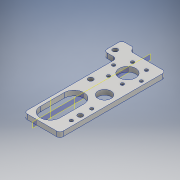
# Autodesk Inventor part: side_plate
Saved by Autodesk Inventor 2018 (Build 220112000, 112)
## iProperties
Created: 2019-01-31
Part Number: side_plate
Material: Aluminum 6061
Document SubType Name: Modeling
Designer: steve
Density: 2.7 g/cm^3
Appearance: Aluminum - Flat
Mass: 11.8642 g
Surface Area: 37.8269 cm^2
Volume: 4.39413 cm^3
d0: 10,000 mm
d1: 10,100 mm
d2: 25,000 mm
d3: 13,000 mm
d4: 15,000 mm
d5: 8,000 mm
d6: 42,800 mm
d7: 45,00 deg
d8: 38,100 mm
d9: 6,000 mm
d10: 2,000 mm
d11: 3,000 mm
d12: 3,000 mm
d13: 3,000 mm
d14: 0,00 deg
d15: 17,000 mm
d16: 6,000 ul
d20: 2,000 mm
d27: 22,000 mm
d28: 12,100 mm
d29: 14,600 mm
d30: 3,000 mm
d31: 2,000 mm
d33: 0,00 deg
d34: 26,000 mm
d35: 14,000 mm
d36: 6,000 mm
d37: 27,000 mm
d38: 3,000 mm
tol: 0,100 mm
z_motor: 50,000 ul
z_roller: 26,000 ul
pitch: 0,500 mm
roller_diam: 15,000 mm
roller_bearing_dia: 8,000 mm
ball_roller_angle: 45,00 deg
absorber_dia: 12,100 mm
absorber_length: 2,500 mm
d18: 360,00 deg
Author: steve
Autodesk Inventor part; units mm, degrees
ref_plane "YZ Plane" through (0, 0, 0) normal (1, 0, 0) x (0, 1, 0)
ref_plane "XZ Plane" through (0, 0, 0) normal (0, 1, 0) x (-1, 0, 0)
ref_plane "XY Plane" through (0, 0, 0) normal (0, 0, 1) x (1, 0, 0)
sketch "Sketch1" plane through (0, 0, 0) normal (0, 0, 1) x (1, 0, 0)
  circle A0 centre (0, 0) radius 5 construction
  circle A1 centre (0, 0) radius 5.05
  line L0 (-11, 12.5) -> (11, 12.5)
  line L1 (11, 12.5) -> (11, -52.3463)
  line L2 (11, -52.3463) -> (-11, -52.3463)
  line L3 (-11, -52.3463) -> (-11, 12.5)
  circle A2 centre (0, 0) radius 12.5 construction
  circle A3 centre (4.5, -18.5109) radius 6.5 construction
  circle A4 centre (4.5, -18.5109) radius 7.5 construction
  circle A5 centre (4.5, -18.5109) radius 4
  circle A6 centre (24.9354, -38.9463) radius 21.4 construction
  line L4 (4.5, -18.5109) -> (24.9354, -38.9463) construction
  line L5 (0, 48.1253) -> (0, -78.4249) construction
  circle A7 centre (0, 0) radius 19.05 construction
  line L6 (54.9772, -60.3463) -> (-51.313, -60.3463) construction
  line L7 (-70.5727, -54.3463) -> (77.7123, -54.3463) construction
  line L8 (8, -57.4182) -> (8, 30.0467) construction
  circle A8 centre (8, -36.8463) radius 1.5
  circle A9 centre (0, 0) radius 11 construction
  line L9 (12, -6.3386) -> (12, -55.2043) construction
  dimension "d8" = 38.1
  dimension "d0" = 10
  dimension "d1" = 10.1
  dimension "d2" = 25
  dimension "d3" = 13
  dimension "d4" = 15
  dimension "d5" = 8
  dimension "d6" = 42.8
  dimension "d7" = 45
  dimension "d9" = 6
  dimension "d10" = 2
  dimension "d11" = 3
  dimension "d12" = 3
  dimension "d27" = 22
  dimension "d71" = 15.5
  dimension "d84" = 64.8463
  dimension "d85" = 1
  constraints: 18 end point, 9 centre point, 7 coincident, 6 tangent, 3 horizontal, 2 parallel, 2 vertical, 1 perpendicular, 1 point on line, 3 other
  measures "d0" diameter of A0
  measures "d1" diameter of A1
  measures "d2" diameter of A2
  measures "d3" diameter of A3
  measures "d4" diameter of A4
  measures "d5" diameter of A5
  measures "d6" diameter of A6
  measures "d7" angle of L5 L4
  measures "d9" distance between parallel lines of L6 L7
  measures "d10" distance between parallel lines of L7 L2
  measures "d11" distance between parallel lines of L1 L8
  measures "d12" diameter of A8
  measures "d27" diameter of A9
  measures "d71" distance from line of A8.centre L2
  measures "d84" distance between parallel lines of L2 L0
  measures "d85" distance between parallel lines of L1 L9
extrude "Extrusion1" add sketch "Sketch1" along normal blind 3
sketch "Sketch2" plane through (0, 0, 0) normal (0, 0, -1) x (-1, 0, 0)
  circle A0 centre (0, 0) radius 8.5 construction
  line L0 (-15.4, 0) -> (15.4, 0) construction
  point P0 (-8.5, 0)
  point P1 (-4.25, -7.3612)
  point P2 (4.25, -7.3612)
  point P3 (8.5, 0)
  point P4 (4.25, 7.3612)
  point P5 (-4.25, 7.3612)
  dimension "d15" = 17
  dimension "d18" = 360
  constraints: 1 coincident, 1 horizontal alignment, 1 point on line, 9 other
hole "Hole1" at (8.5, 0, 0) at (4.25, -7.3612, 0) at (-4.25, -7.3612, 0) at (-8.5, 0, 0) at (-4.25, 7.3612, 0) at (4.25, 7.3612, 0) direction (0, 0, 1) diameter 2 end through all counterbore diameter 4 counterbore depth 2
sketch "Sketch3" plane through (0, 0, 3) normal (0, 0, 1) x (1, 0, 0)
  circle A0 centre (-3, -29.6963) radius 6.05 construction
  circle A1 centre (-3, -44.2963) radius 6.05 construction
  line L0 (-3, -52.9991) -> (-3, -16.007) construction
  line L1 (0, 25.5998) -> (0, -66.099) construction
  line L2 (-19.4661, -50.3463) -> (34.3963, -50.3463) construction
  line L3 (-11, -52.3463) -> (11, -52.3463) construction
  line L4 (-9.05, -29.6963) -> (-9.05, -44.2963)
  line L5 (3.05, -29.6963) -> (3.05, -44.2963)
  arc A2 (3.05, -29.6963) -> (-9.05, -29.6963) centre (-3, -29.6963) ccw
  arc A3 (-9.05, -44.2963) -> (3.05, -44.2963) centre (-3, -44.2963) ccw
  point P0 (0, 0)
  dimension "d28" = 12.1
  dimension "d29" = 14.6
  dimension "d30" = 3
  dimension "d31" = 2
  constraints: 8 end point, 8 point on circle, 4 centre point, 3 tangent, 3 vertical, 2 coincident, 2 point on line, 1 equal radius, 1 horizontal
  measures "d28" diameter of A0
  measures "d29" distance of A0.centre A1.centre
  measures "d30" distance between parallel lines of L0 L1
  measures "d31" distance between parallel lines of L3 L2
extrude "Extrusion2" cut sketch "Sketch3" against normal through all
sketch "Sketch4" plane through (0, 0, 3) normal (0, 0, 1) x (1, 0, 0)
  circle A0 centre (0, 0) radius 13 construction
  circle A1 centre (4.5, -18.5109) radius 4 construction
  circle A2 centre (4.5, -18.5109) radius 7 construction
  line L0 (-30.9627, -14.5) -> (22.7085, -14.5) construction
  line L1 (-11, 12.5) -> (-11, -52.3463) construction
  line L2 (11, 12.5) -> (-11, 12.5) construction
  line L3 (-11, -12.7679) -> (-8, -11.0359) construction
  line L4 (-8, -11.0359) -> (-5, -12.7679) construction
  line L5 (-5, -12.7679) -> (-5, -16.2321) construction
  line L6 (-5, -16.2321) -> (-8, -17.9641) construction
  line L7 (-8, -17.9641) -> (-11, -16.2321) construction
  line L8 (-11, -16.2321) -> (-11, -12.7679) construction
  circle A3 centre (-8, -14.5) radius 2.8 construction
  dimension "d34" = 26
  dimension "d35" = 14
  dimension "d36" = 6
  dimension "d37" = 27
  dimension "d72" = 5.6
  constraints: 14 end point, 4 coincident, 3 centre point, 2 collinear, 1 horizontal, 1 point on line, 13 other
  measures "d34" diameter of A0
  measures "d35" diameter of A2
  measures "d36" distance between parallel lines of L6 L3
  measures "d37" distance from line of L2 point (-8, -14.5)
  measures "d72" diameter of A3
hole "Hole2" at (-8, -14.5, 3) direction (0, 0, -1) diameter 3 end through all
ref_plane "Work Plane1" through (-3, -29.6963, 3) normal (-1, 0, 0) x (0, 0, -1)
sketch "Sketch8" plane through (0, 0, 3) normal (0, 0, 1) x (1, 0, 0)
  line L0 (11, 12.5) -> (-11, 12.5) projected
  line L1 (-11, 12.5) -> (-19, 12.5)
  line L2 (-19, 12.5) -> (-19, 4.5)
  line L3 (-19, 4.5) -> (-11, 4.5)
  line L4 (-11, 4.5) -> (-11, 12.5)
  point P0 (0, 0)
  dimension "d58" = 8
  dimension "d59" = 8
  constraints: 8 end point, 2 parallel, 1 horizontal, 1 perpendicular
  measures "d58" distance of L0.end L1.end
  measures "d59" distance of L1.end L2.end
extrude "Extrusion4" add sketch "Sketch8" against normal up to surface (3 mm away)
sketch "Sketch9" plane through (0, 0, 3) normal (0, 0, 1) x (1, 0, 0)
  line L0 (-19, 12.5) -> (-19, 4.5) construction
  line L1 (-19, 8.5) -> (-9.7013, 8.5) construction
  line L2 (11, 12.5) -> (-19, 12.5) construction
  line L3 (-16, 12.5) -> (-16, 1.2197) construction
  point P0 (0, 0)
  point P1 (-16, 8.5)
  dimension "d62" = 3
  constraints: 4 end point, 3 point on line, 1 horizontal, 1 midpoint, 1 vertical
  measures "d62" distance between parallel lines of L0 L3
hole "Hole4" at (-16, 8.5, 3) direction (0, 0, -1) diameter 3 end through all
fillet "Fillet2" radius 2 6 edges at (11, -52.3463, 1.5) (-11, -52.3463, 1.5) (11, 12.5, 1.5) (-19, 12.5, 1.5) (-19, 4.5, 1.5) (-11, 4.5, 1.5)
sketch "Sketch12" plane through (0, 0, 3) normal (0, 0, 1) x (1, 0, 0)
  circle A0 centre (8, -36.8463) radius 1.5 construction
  line L0 (8, -27.4514) -> (8, -47.8605) construction
  line L1 (24.4744, -26.8463) -> (0, -26.8463) construction
  line L2 (-0.5807, -45.3463) -> (23.4788, -45.3463) construction
  line L3 (0.6637, -29.8463) -> (21.6536, -29.8463) construction
  line L4 (0, -42.3463) -> (23.4788, -42.3463) construction
  point P0 (0, 0)
  point P1 (8, -29.8463)
  point P2 (8, -42.3463)
  dimension "d73" = 10
  dimension "d74" = 8.5
  dimension "d75" = 3
  dimension "d76" = 3
  constraints: 10 end point, 5 point on line, 4 horizontal, 1 vertical
  measures "d73" distance from line of L1 A0.centre
  measures "d74" distance from line of A0.centre L2
  measures "d75" distance between parallel lines of L1 L3
  measures "d76" distance between parallel lines of L4 L2
hole "Hole5" at (8, -29.8463, 3) at (8, -42.3463, 3) direction (0, 0, -1) diameter 2.013 end through all thread size "M2.5x0.45" class "6H" standard "ANSI Metric M Profile"
sketch "Sketch13" plane through (0, 0, 3) normal (0, 0, 1) x (1, 0, 0)
  line L0 (-19, 10.5) -> (-19, 6.5) construction
  line L1 (9, 12.5) -> (-17, 12.5) construction
  line L2 (-19, 10.5) -> (-19, 15.5)
  line L3 (-19, 15.5) -> (-11, 15.5)
  line L4 (-11, 15.5) -> (-11, 12.5)
  line L5 (-11, 2.5) -> (-11, -50.3463) projected
  arc A0 (-17, 12.5) -> (-19, 10.5) centre (-17, 10.5) ccw projected
  line L6 (-17, 12.5) -> (-11, 12.5)
  point P0 (0, 0)
  dimension "d86" = 3
  constraints: 8 end point, 2 collinear, 2 perpendicular, 1 point on line, 1 vertical
  measures "d86" distance between parallel lines of L3 L1
extrude "Extrusion5" add sketch "Sketch13" against normal up to surface (3 mm away)
fillet "Fillet3" radius 2 3 edges at (-19, 15.5, 1.5) (-11, 15.5, 1.5) (-11, 12.5, 1.5)
equation "\"d8\" = d2 + d3 + tol"
equation "\"d4\" = roller_diam"
equation "\"d5\" = roller_bearing_dia"
equation "\"d7\" = ball_roller_angle"
equation "\"d28\" = absorber_dia"
equation "\"d29\" = absorber_dia + absorber_length"
equation "\"tol\" = 0.1"
equation "\"z_motor\" = 50"
equation "\"z_roller\" = 26"
equation "\"pitch\" = 0.5"
equation "\"roller_diam\" = 15"
equation "\"roller_bearing_dia\" = 8"
equation "\"ball_roller_angle\" = 45deg"
equation "\"absorber_dia\" = 12.1"
equation "\"absorber_length\" = 2.5"
body "Solid1"
